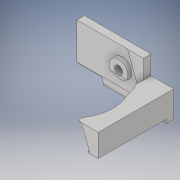
# Autodesk Inventor part: finger_root_plate
Saved by Autodesk Inventor 2019 (Build 230136000, 136)
## iProperties
Created: 2024-08-26
Part Number: finger_root_plate
Material: Generisch
Document SubType Name: Modeling
Designer: nic
Density: 1 g/cm^3
Appearance: Vorgabe
Author: nic
Autodesk Inventor part; units mm, degrees
ref_plane "YZ Plane" through (0, 0, 0) normal (1, 0, 0) x (0, 1, 0)
ref_plane "XZ Plane" through (0, 0, 0) normal (0, 1, 0) x (-1, 0, 0)
ref_plane "XY Plane" through (0, 0, 0) normal (0, 0, 1) x (1, 0, 0)
ref_plane "Arbeitsebene1" through (0, 0, -3.5) normal (0, 0, 1) x (1, 0, 0)
sketch "Skizze2" plane through (0, 0, -3.5) normal (0, 0, 1) x (1, 0, 0)
  circle A0 centre (-4.2286, -1.5391) radius 0.8222 construction
  circle A1 centre (-4.2286, -1.5391) radius 1.1
  circle A2 centre (-4.2286, -1.5391) radius 2.5
  point P0 (0, 0)
  dimension "d0" = 2.2
  dimension "d1" = 5
  constraints: 2 centre point, 2 coincident
  measures "d0" diameter of A1
  measures "d1" diameter of A2
extrude "Extrusion1" add sketch "Skizze2" against normal blind 2
sketch "Skizze3" plane through (0, 0, 0) normal (1, 0, 0) x (0, 1, 0)
  line L0 (-4.0391, -5.5) -> (0.9609, -5.5) construction
  line L1 (-4.0391, -3.5) -> (0.9609, -3.5) construction
  line L2 (-5.8067, -4.3839) -> (-3.1169, -3.5722) construction
  line L3 (-3.1169, -3.5722) -> (-2.3455, -3.3472) construction
  line L4 (-4.0391, -3.5) -> (-4.0391, -5.5) projected
  line L5 (-4.0391, -3.8505) -> (-4.0391, -4.1505)
  line L6 (-4.0391, -4.1505) -> (-2.6391, -3.5)
  line L7 (-2.6391, -3.5) -> (-2.6391, -5.5) projected
  line L8 (-4.0391, -3.8505) -> (-4.0391, -3.5)
  line L9 (-4.0391, -3.5) -> (0.9609, -3.5) projected
  line L10 (-2.6391, -3.5) -> (-4.0391, -3.5)
  point P0 (0, 0)
  dimension "d4" = 0.3
  constraints: 8 end point, 6 point on line, 2 collinear
  measures "d4" distance of L5.start L5.end
extrude "Extrusion2" cut sketch "Skizze3" against normal through all
sketch "Skizze4" plane through (-4.2286, -1.5391, -5.5) normal (0, 0, -1) x (-1, 0, 0)
  circle A0 centre (0, 0) radius 1.1 projected
  line L0 (0, 0) -> (0, -6) construction
  line L1 (5.6101, 6) -> (-5.6101, 6)
  line L2 (-5.6101, 6) -> (-5.6101, -6)
  line L3 (-5.6101, -6) -> (5.6101, -6)
  line L4 (5.6101, -6) -> (5.6101, 6)
  line L5 (5.6101, 6) -> (-5.6101, -6) construction
  line L6 (-5.6101, 6) -> (5.6101, -6) construction
  line L7 (0, 0) -> (0, 5)
  line L8 (-5.6101, 5) -> (5.6101, 5)
  point P0 (-4.2286, 1.5391)
  dimension "d7" = 6
  dimension "d8" = 5
  constraints: 18 end point, 2 midpoint, 2 parallel, 2 perpendicular, 2 point on line, 2 vertical, 1 horizontal
  measures "d7" distance of L0.start L0.end
  measures "d8" distance of L0.start L7.end
extrude "Extrusion3" add sketch "Skizze4" along normal mid plane 2 contours L4 L3 L2 L8
sketch "Skizze5" plane through (-4.2286, -1.5391, -6.5) normal (0, 0, -1) x (-1, 0, 0)
  circle A0 centre (0, 0) radius 1.1 construction
  line L0 (12, 0) -> (12, 5)
  line L1 (12, 5) -> (0, 5)
  line L2 (0, 5) -> (0, 1.1)
  line L3 (12, 0) -> (12, -5.1)
  line L4 (12, -5.1) -> (0, -5.1)
  line L5 (0, -5.1) -> (0, -1.1)
  arc A1 (0, -1.1) -> (0, 1.1) centre (0, 0) ccw
  line L6 (0, 5) -> (12, 5)
  line L7 (12, 5) -> (12, -5.1)
  line L8 (12, -5.1) -> (0, -5.1)
  line L9 (0, -5.1) -> (0, -1.1)
  line L10 (0, 1.1) -> (0, 5)
  point P0 (-4.2286, 1.5391)
  constraints: 22 end point, 5 parallel, 4 point on circle, 1 centre point, 1 coincident, 1 concentric, 1 horizontal, 1 perpendicular
extrude "Extrusion5" add sketch "Skizze5" against normal up to surface (2 mm away)
sketch "Skizze6" plane through (-4.2286, -1.5391, -6.5) normal (0, 0, -1) x (-1, 0, 0)
  line L0 (12, 5) -> (-5.6101, 5) construction
  line L1 (-5.6101, 5) -> (-5.6101, -6) construction
  line L2 (-5.6101, -6) -> (5.6101, -6) construction
  line L3 (5.6101, -6) -> (5.6101, -5.1) construction
  line L4 (5.6101, -5.1) -> (12, -5.1) construction
  line L5 (12, -5.1) -> (12, 5) construction
  circle A0 centre (0, 0) radius 1.1 construction
  line L6 (-5.6101, -6) -> (-11.6202, -6)
  line L7 (-11.6202, -6) -> (-11.6202, 0)
  line L8 (-11.6202, 0) -> (-5.6101, 0)
  line L9 (-5.6101, 0) -> (-5.6101, -6)
  point P0 (-4.2286, 1.5391)
  constraints: 8 end point, 2 parallel, 1 horizontal, 1 perpendicular
extrude "Extrusion6" add sketch "Skizze6" against normal blind 20
ref_plane "Arbeitsebene2" through (2.9294, -0.9766, 3.8598) normal (-0.3583676, 0.9335804, -0.0005065) x (-0.0014134, 0, 0.999999)
sketch "Skizze8" plane through (2.9294, -0.9766, 3.8598) normal (-0.3583676, 0.9335804, -0.0005065) x (-0.0014134, 0, 0.999999)
  line L0 (-4.0194, -1.3576) -> (0, 0) construction
  line L1 (0, 0) -> (4.2744, 0) construction
  line L2 (4.2744, 0) -> (8.2939, -1.3576) construction
  arc A0 (8.2939, -1.3576) -> (-4.0194, -1.3576) centre (2.1372, -10.893) ccw construction
  arc A1 (8.959, -1.5726) -> (-4.7092, -1.5906) centre (2.1372, -10.893) ccw
  line L3 (-4.7092, -1.5906) -> (8.959, -1.5726)
  line L4 (-8.3576, -3.8079) -> (9.6424, -3.7842) projected
  point P0 (-3.8557, -2.3899)
  constraints: 4 point on circle, 2 centre point, 2 end point, 1 parallel
extrude "Extrusion7" cut sketch "Skizze8" against normal blind 20
ref_plane "Arbeitsebene4" through (2.9294, -0.9766, 3.8598) normal (-0.3583676, 0.9335804, -0.0005065) x (-0.0014134, 0, 0.999999)
sketch "Skizze10" plane through (2.9294, -0.9766, 3.8598) normal (-0.3583676, 0.9335804, -0.0005065) x (-0.0014134, 0, 0.999999)
  arc A0 (8.955, -1.5696) -> (-4.6806, -1.5696) centre (2.1372, -10.893) ccw projected
  line L0 (-8.3576, -3.8079) -> (9.6424, -3.7842) projected
  arc A1 (-2.9419, -0.5195) -> (-8.3576, -3.8079) centre (-2.6067, -7.1753) ccw
  line L1 (-8.3576, -3.8079) -> (-2.9419, -0.5195)
  point P0 (-3.8557, -2.3899)
  constraints: 3 point on circle, 2 end point, 1 centre point
extrude "Extrusion8" cut sketch "Skizze10" against normal blind 20
sketch "Skizze12" plane through (-9.8387, -7.5391, -6.5) normal (-1, 0, 0) x (0, 0, 1)
  line L0 (2, 0.9) -> (2, 0) projected
  line L1 (2, 0) -> (0, 0)
  line L2 (0, 0) -> (0, -1)
  line L3 (0, -1) -> (2, -1)
  line L4 (2, -1) -> (2, 0)
  point P0 (6.5, 7.5391)
  dimension "d24" = 1
  constraints: 8 end point, 2 parallel, 1 horizontal, 1 perpendicular
  measures "d24" distance of L2.end L1.end
extrude "Extrusion9" add sketch "Skizze12" against normal up to surface (17.2303 mm away)
sketch "Skizze13" plane through (-16.2286, -6.6391, -6.5) normal (-1, 0, 0) x (0, 0, 1)
  line L0 (1.6586, -1.4704) -> (1.4677, -3.7755) projected
  line L1 (1.6586, -1.4704) -> (2.1161, 0.8323) projected
  line L2 (2.1161, 0.8323) -> (2.9278, 3.5222) projected
  line L3 (0, -1.9) -> (2, -1.9) projected
  line L4 (2, -0.9) -> (2, 5.1) projected
  line L5 (1.623, -1.9) -> (2, -1.9) construction
  line L6 (2, -1.9) -> (2, 0.2478) construction
  line L7 (2, 0.2478) -> (1.9398, 0.2478)
  line L8 (1.623, -1.6495) -> (1.623, -1.9) construction
  line L9 (1.623, -1.6495) -> (1.9398, 0.2478) construction
  line L10 (1.423, -2.1) -> (2.2, -2.1)
  line L11 (2.2, -2.1) -> (2.2, 0.4478)
  line L12 (2.2, 0.4478) -> (1.7704, 0.4478)
  line L13 (1.7704, 0.4478) -> (1.423, -1.6329)
  line L14 (1.423, -1.6329) -> (1.423, -2.1)
  point P0 (6.5, 6.6391)
  dimension "d27" = 0.2
  constraints: 20 end point, 6 point on line, 4 parallel, 2 perpendicular, 1 horizontal, 4 other
  measures "d27" distance between parallel lines of L8 L14
extrude "Extrusion10" cut sketch "Skizze13" against normal up to surface (17.6101 mm away)
sketch "Skizze14" plane through (2.9294, -0.9766, 3.8598) normal (-0.3583676, 0.9335804, -0.0005065) x (-0.0014134, 0, 0.999999)
  arc A0 (-6.3588, -1.6677) -> (-8.3576, -3.8079) centre (-2.6067, -7.1753) ccw construction
  arc A1 (-2.9419, -0.5195) -> (-6.2107, -1.5696) centre (-2.6067, -7.1753) ccw construction
  line L0 (-8.3576, -3.8079) -> (9.6424, -3.7842) construction
  arc A2 (8.955, -1.5696) -> (-2.9419, -0.5195) centre (2.1372, -10.893) ccw construction
  line L1 (9.6424, -1.634) -> (9.6424, -3.7842) construction
  line L2 (8.955, -1.5696) -> (-6.2107, -1.5696) construction
  line L3 (-8.3576, -1.6577) -> (9.6424, -1.634) construction
  line L4 (8.955, -4.108) -> (-6.2107, -4.108)
  line L5 (-6.2107, -1.5696) -> (8.955, -1.5696)
  line L6 (8.955, -1.5696) -> (8.955, -4.108)
  line L7 (-8.3576, -3.8079) -> (-6.2107, -2.5043)
  line L8 (-8.3576, -3.8079) -> (-4.706, -1.5906) construction
  line L9 (-8.3576, -3.8079) -> (-6.2107, -4.108)
  line L10 (-6.2107, -2.5043) -> (-6.2107, -1.5696)
  point P0 (-3.8557, -2.3899)
  constraints: 12 end point, 2 parallel, 1 horizontal, 1 perpendicular, 1 point on line
extrude "Extrusion11" cut sketch "Skizze14" along normal through all both and the other way through all
sketch "Skizze15" plane through (1.3815, -1.5391, -6.5) normal (0, 1, 0) x (1, 0, 0)
  line L0 (-0.0096, -4.1555) -> (0.0913, -4.1555)
  line L1 (0.0913, -4.1555) -> (0.0913, -4.1471)
  line L2 (-0.0096, -3.9833) -> (-0.0096, -4.1555)
  ellipse E0 centre (-5.1471, -7.7437) end of major axis (-5.1377, -1.0794) minor radius 6.2216 (0.0913, -4.1471) -> (0, -3.9988) ccw construction
  line L3 (0.0913, -4.1471) -> (-0.0096, -3.9838)
  point P0 (-1.3815, -6.5)
  point P1 (0, -4.1469)
  constraints: 8 end point, 1 horizontal, 1 parallel, 1 perpendicular, 1 point on line, 2 other
extrude "Extrusion12" cut sketch "Skizze15" against normal up to surface surface through (2.066, -1.3069, 5.9827) normal (-0.3583676, 0.9335804, -0.0005065)
sketch "Skizze16" plane through (-4.2286, -1.5391, 13.5) normal (0, 0, 1) x (1, 0, 0)
  line L0 (7.8732, -5.318) -> (8.1404, -6.7324) construction
  line L1 (5.6772, -0.0011) -> (7.98, -6) construction
  line L2 (5.6101, 0) -> (5.6101, -6) construction
  arc A0 (7.98, -6) -> (5.6101, -0.6327) centre (-4.9774, -8.5144) ccw construction
  line L3 (5.6101, -6) -> (11.6202, -6) construction
  line L4 (7.98, -6) -> (5.6101, -6) construction
  line L5 (5.6101, -6) -> (5.6101, -0.6327) construction
  arc A1 (8.1007, -6.1) -> (5.5101, -0.3365) centre (-4.9774, -8.5144) ccw
  line L6 (8.1007, -6.1) -> (5.5101, -6.1)
  line L7 (5.5101, -6.1) -> (5.5101, -0.3365)
  point P0 (4.2286, 1.5391)
  dimension "d36" = 0.1
  constraints: 8 end point, 4 point on circle, 2 centre point, 2 collinear, 1 point on line, 2 other
  measures "d36" radial gap between concentric circles of A0 A1
extrude "Extrusion14" cut sketch "Skizze16" against normal blind 2
fillet "Rundung1" radius 3 1 edges at (3.1175, -5.0538, 12.3916)
fillet "Rundung2" radius 1 3 edges at (3.2083, -5.2837, 13.5) (3.8021, -7.2824, 13.5) (1.9295, -2.7498, 13.5)
